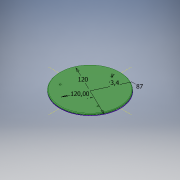
# Autodesk Inventor part: Base-Plate
Saved by Autodesk Inventor 2018.2 (Build 222227000, 227)
## iProperties
Created: 2018-02-19
Part Number: Base-Plate
Material: Generisch
Document SubType Name: Modeling
Designer: JochenAlt
Density: 1 g/cm^3
Appearance: Vorgabe
Author: JochenAlt
Autodesk Inventor part; units mm, degrees
ref_plane "YZ Plane" through (0, 0, 0) normal (1, 0, 0) x (0, 1, 0)
ref_plane "XZ Plane" through (0, 0, 0) normal (0, 1, 0) x (-1, 0, 0)
ref_plane "XY Plane" through (0, 0, 0) normal (0, 0, 1) x (1, 0, 0)
sketch "Skizze1" plane through (0, 0, 0) normal (0, 0, 1) x (1, 0, 0)
  circle A0 centre (0, 0) radius 60
  circle A1 centre (0, 0) radius 43.5 construction
  circle A2 centre (0, 43.5) radius 1.7
  circle A3 centre (37.6721, -21.75) radius 1.7
  circle A4 centre (-37.6721, -21.75) radius 1.7
  line L0 (0, 0) -> (37.6721, -21.75) construction
  line L1 (0, 0) -> (-37.6721, -21.75) construction
  line L2 (0, 84) -> (0, -84) construction
  line L3 (-84, 0) -> (84, 0) construction
  dimension "d0" = 120
  dimension "d1" = 87
  dimension "d2" = 3.4
  dimension "d3" = 120
  constraints: 5 centre point, 4 end point, 3 point on circle, 2 coincident, 2 equal radius, 1 symmetric about line
  measures "d0" diameter of A0
  measures "d1" diameter of A1
  measures "d2" diameter of A2
  measures "d3" angle of L1 L0
extrude "Extrusion1" add sketch "Skizze1" along normal blind 3
fillet "Rundung1" radius 1 2 edges at (-60, 0, 3) (-60, 0, 0)
